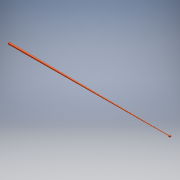
# Autodesk Inventor part: STACER
Saved by Autodesk Inventor 2016 (Build 200138000, 138)
## iProperties
Created: 2016-01-01
Part Number: STACER
Material: Generic
Document SubType Name: Modeling
Designer: jonathan
Density: 1 g/cm^3
Appearance: Copper - Polished
Author: jonathan
Autodesk Inventor part; units mm, degrees
ref_plane "XZ Plane" through (0, 0, 0) normal (0, 1, 0) x (-1, 0, 0)
ref_plane "XY Plane" through (0, 0, 0) normal (0, 0, 1) x (1, 0, 0)
sketch "Sketch1" plane through (0, 0, 0) normal (1, 0, 0) x (0, 1, 0)
  circle A0 centre (0, 0) radius 10
  dimension "d0" = 20
  constraints: 1 centre point, 1 coincident
  measures "d0" diameter of A0
ref_plane "Work Plane1" through (1500, 0, 0) normal (1, 0, 0) x (0, 1, 0)
sketch "Sketch2" plane through (1500, 0, 0) normal (1, 0, 0) x (0, 1, 0)
  circle A0 centre (0, 0) radius 2.5
  dimension "d2" = 5
  constraints: 1 centre point, 1 coincident
  measures "d2" diameter of A0
loft "Loft1" add profiles "Sketch1", "Sketch2"
sketch "Sketch3" plane through (1500, 0, 0) normal (1, 0, 0) x (0, 0, -1)
  circle A0 centre (0, 0) radius 10
  line L0 (0, 10) -> (0, -10)
  dimension "d7" = 20
  dimension "d8" = 0
  constraints: 2 end point, 2 point on circle, 1 centre point, 1 coincident, 1 vertical
  measures "d7" diameter of A0
  measures "d8" distance from line of point (0, 0) L0
revolve "Revolution1" add sketch "Sketch3" angle 360 about axis through (1500, 10, 0) along (0, -1, 0) picked at (-1.5491, -2.9515) contours L0 A0
body "Solid1"
